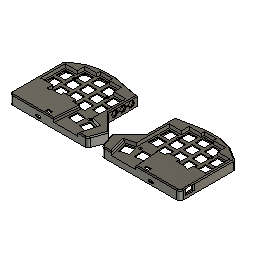
top_23332_2 (Autodesk Fusion 360 design; units mm, degrees)
Autodesk Fusion 360 part; units mm, degrees
note: some values were not read from the file. Set by a fixed rule: which sketch regions a step uses.
sketch "case_plate_23332_2" plane through (0, 0, 0) normal (0, 0, 1) x (1, 0, 0)
  line L0 (-131.5, 89.0512) -> (-131.5, 7.28)
  line L1 (-131.5, 7.28) -> (-13.7052, 7.28)
  line L2 (-32.5, 98.826) -> (-72.3112, 106.482)
  line L3 (-91.6231, 106.5) -> (-111.8983, 101.4312)
  line L4 (-13.7052, 7.28) -> (-6.0652, 28.2707)
  line L5 (-72.3112, 106.482) -> (-72.4047, 106.5)
  line L6 (-72.4047, 106.5) -> (-91.6231, 106.5)
  line L7 (-6.0652, 28.2707) -> (-32.5, 54.6647)
  line L8 (-32.5, 54.6647) -> (-32.5, 98.826)
  line L9 (-111.8983, 101.4312) -> (-131.5, 89.0512)
  line L10 (-29.5, 101.3041) -> (-72.1189, 109.5)
  line L11 (-91.9924, 109.5) -> (-113.0931, 104.2248)
  line L12 (-2.5919, 29.0421) -> (-29.5, 55.9087)
  line L13 (-134.5, 90.7047) -> (-134.5, 4.28)
  line L14 (-11.6046, 4.28) -> (-2.5919, 29.0421)
  line L15 (-134.5, 4.28) -> (-11.6046, 4.28)
  line L16 (-72.1189, 109.5) -> (-91.9924, 109.5)
  line L17 (-113.0931, 104.2248) -> (-134.5, 90.7047)
  line L18 (-29.5, 55.9087) -> (-29.5, 101.3041)
  line L19 (-112.3762, 102.5487) -> (-132.7, 89.7126)
  line L20 (-12.865, 6.08) -> (-4.6759, 28.5793)
  line L21 (-31.3, 99.8172) -> (-72.2904, 107.7)
  line L22 (-4.6759, 28.5793) -> (-31.3, 55.1623)
  line L23 (-91.7708, 107.7) -> (-112.3762, 102.5487)
  line L24 (-132.7, 89.7126) -> (-132.7, 6.08)
  line L25 (-31.3, 55.1623) -> (-31.3, 99.8172)
  line L26 (-132.7, 6.08) -> (-12.865, 6.08)
  line L27 (-72.2904, 107.7) -> (-91.7708, 107.7)
  line L28 (-12.4448, 5.48) -> (-3.9812, 28.7336)
  line L29 (-112.6152, 103.1074) -> (-133.3, 90.0433)
  line L30 (-133.3, 90.0433) -> (-133.3, 5.48)
  line L31 (-91.8447, 108.3) -> (-112.6152, 103.1074)
  line L32 (-72.2332, 108.3) -> (-91.8447, 108.3)
  line L33 (-30.7, 100.3128) -> (-71.9712, 108.2496)
  line L34 (-133.3, 5.48) -> (-12.4448, 5.48)
  line L35 (-3.9812, 28.7336) -> (-30.7, 55.4111)
  line L36 (-30.7, 55.4111) -> (-30.7, 100.3128)
  line L37 (-71.9712, 108.2496) -> (-72.2332, 108.3)
  circle A0 centre (-108, 80.5) radius 2.2
  circle A1 centre (-56, 80.5) radius 2.2
  circle A2 centre (-39.8644, 36.6759) radius 2.2
  line L38 (-96.5, 10.39) -> (-96.5, 28.39)
  line L39 (-96.5, 28.39) -> (-129.5, 28.39)
  line L40 (-129.5, 10.39) -> (-96.5, 10.39)
  line L41 (-129.5, 28.39) -> (-129.5, 10.39)
  line L42 (-92.975, 13.01) -> (-92.975, 7.16)
  line L43 (-84.175, 7.16) -> (-84.175, 13.01)
  line L44 (-84.175, 13.01) -> (-92.975, 13.01)
  line L45 (-82.175, 12.025) -> (-82.175, 8.525)
  line L46 (-73.175, 8.525) -> (-73.175, 12.025)
  line L47 (-73.175, 12.025) -> (-82.175, 12.025)
  line L48 (-82.175, 8.525) -> (-73.175, 8.525)
  line L49 (-17.3936, 37.8282) -> (-25.1718, 45.6064)
  line L50 (-25.1718, 45.6064) -> (-31.6064, 39.1718)
  line L51 (-21.0041, 34.2177) -> (-17.3936, 37.8282)
  line L52 (-96.8, 31.55) -> (-96.8, 40.45)
  line L53 (-96.8, 40.45) -> (-104.8004, 40.45)
  line L54 (-105.4, 39.7287) -> (-105.4, 31.55)
  line L55 (-105.4, 31.55) -> (-96.8, 31.55)
  line L56 (-127, 52) -> (-113, 52)
  line L57 (-113, 66) -> (-127, 66)
  line L58 (-127, 66) -> (-127, 52)
  line L59 (-113, 52) -> (-113, 66)
  line L60 (-127, 71) -> (-113, 71)
  line L61 (-113, 71) -> (-113, 85)
  line L62 (-127, 85) -> (-127, 71)
  line L63 (-113, 85) -> (-127, 85)
  line L64 (-108, 59) -> (-108, 45)
  line L65 (-94, 45) -> (-94, 59)
  line L66 (-94, 59) -> (-108, 59)
  line L67 (-108, 45) -> (-94, 45)
  line L68 (-94, 64) -> (-94, 78)
  line L69 (-94, 78) -> (-108, 78)
  line L70 (-108, 78) -> (-108, 64)
  line L71 (-108, 64) -> (-94, 64)
  line L72 (-108, 83) -> (-94, 83)
  line L73 (-94, 83) -> (-94, 97)
  line L74 (-108, 97) -> (-108, 83)
  line L75 (-94, 97) -> (-108, 97)
  line L76 (-89, 50) -> (-75, 50)
  line L77 (-75, 64) -> (-89, 64)
  line L78 (-75, 50) -> (-75, 64)
  line L79 (-89, 64) -> (-89, 50)
  line L80 (-89, 83) -> (-89, 69)
  line L81 (-89, 69) -> (-75, 69)
  line L82 (-75, 69) -> (-75, 83)
  line L83 (-75, 83) -> (-89, 83)
  line L84 (-75, 88) -> (-75, 102)
  line L85 (-75, 102) -> (-89, 102)
  line L86 (-89, 88) -> (-75, 88)
  line L87 (-89, 102) -> (-89, 88)
  line L88 (-70, 59) -> (-70, 45)
  line L89 (-56, 45) -> (-56, 59)
  line L90 (-70, 45) -> (-56, 45)
  line L91 (-56, 59) -> (-70, 59)
  line L92 (-70, 64) -> (-56, 64)
  line L93 (-56, 78) -> (-70, 78)
  line L94 (-70, 78) -> (-70, 64)
  line L95 (-56, 64) -> (-56, 78)
  line L96 (-56, 97) -> (-70, 97)
  line L97 (-70, 83) -> (-56, 83)
  line L98 (-70, 97) -> (-70, 83)
  line L99 (-56, 83) -> (-56, 97)
  line L100 (-37, 66) -> (-51, 66)
  line L101 (-51, 52) -> (-37, 52)
  line L102 (-37, 52) -> (-37, 66)
  line L103 (-51, 66) -> (-51, 52)
  line L104 (-51, 71) -> (-37, 71)
  line L105 (-51, 85) -> (-51, 71)
  line L106 (-37, 71) -> (-37, 85)
  line L107 (-37, 85) -> (-51, 85)
  line L108 (-59.7995, 22.3659) -> (-45.8527, 21.1457)
  line L109 (-45.8527, 21.1457) -> (-44.6325, 35.0924)
  line L110 (-58.5793, 36.3126) -> (-59.7995, 22.3659)
  line L111 (-44.6325, 35.0924) -> (-58.5793, 36.3126)
  line L112 (-35.9254, 33.5571) -> (-39.5489, 20.0342)
  line L113 (-39.5489, 20.0342) -> (-26.0259, 16.4107)
  line L114 (-26.0259, 16.4107) -> (-22.4025, 29.9337)
  line L115 (-22.4025, 29.9337) -> (-35.9254, 33.5571)
  line L116 (-131.5, 49.25) -> (-110.75, 49.25)
  line L117 (-129.75, 49.25) -> (-129.75, 87.75)
  line L118 (-110.75, 87.75) -> (-129.75, 87.75)
  line L119 (-91.25, 42.25) -> (-91.25, 47.25)
  line L120 (-110.75, 49.25) -> (-110.75, 42.25)
  line L121 (-91.75, 99.75) -> (-110.75, 99.75)
  line L122 (-110.75, 99.75) -> (-110.75, 87.75)
  line L123 (-91.25, 47.25) -> (-72.75, 47.25)
  line L124 (-72.25, 99.75) -> (-72.25, 104.75)
  line L125 (-72.25, 104.75) -> (-91.75, 104.75)
  line L126 (-91.75, 104.75) -> (-91.75, 99.75)
  line L127 (-72.75, 42.25) -> (-60.8203, 42.25)
  line L128 (-72.75, 47.25) -> (-72.75, 42.25)
  line L129 (-53.25, 87.75) -> (-53.25, 99.75)
  line L130 (-53.25, 99.75) -> (-72.25, 99.75)
  line L131 (-34.25, 54.6647) -> (-34.25, 87.75)
  line L132 (-34.25, 87.75) -> (-53.25, 87.75)
  line L133 (-62.7787, 19.866) -> (-43.1315, 18.1471)
  line L134 (-64.1423, 4.28) -> (-60.8203, 42.25)
  line L135 (-43.1315, 18.1471) -> (-24.0814, 13.0427)
  line L136 (-26.4293, 4.28) -> (-19.0344, 31.8782)
  line L137 (-34.25, 35.9552) -> (-6.2465, 28.4517)
  line L138 (-32.5, 54.6647) -> (-34.25, 54.6647)
  arc A3 (-108, 40.3) -> (-105.8143, 42.25) centre (-108, 42.5) ccw
  line L139 (-105.8143, 42.25) -> (-91.25, 42.25)
  line L140 (-131.5, 47.65) -> (-112.35, 47.65)
  line L141 (-112.35, 47.65) -> (-112.35, 40.65)
  line L142 (-104.6807, 40.65) -> (-89.65, 40.65)
  line L143 (-89.65, 40.65) -> (-89.65, 45.65)
  line L144 (-89.65, 45.65) -> (-74.35, 45.65)
  line L145 (-74.35, 45.65) -> (-74.35, 40.65)
  line L146 (-74.35, 40.65) -> (-62.5664, 40.65)
  line L147 (-34.25, 35.9552) -> (-34.25, 54.6647)
  line L148 (-32.5, 37.298) -> (-32.5, 54.6647)
  line L149 (-65.4859, 7.28) -> (-62.5664, 40.65)
  line L150 (-32.5, 37.298) -> (-8.7266, 30.928)
  line L151 (-31.6064, 39.1718) -> (-28.7198, 36.2851)
  line L152 (-108, 40.3) -> (-110.75, 40.3)
  line L153 (-110.75, 40.3) -> (-110.75, 42.25)
  line L154 (-65.7484, 4.28) -> (-62.5664, 40.65)
  line L155 (-74.35, 40.65) -> (-62.5664, 40.65)
  line L156 (-74.35, 45.65) -> (-74.35, 40.65)
  line L157 (-89.65, 45.65) -> (-74.35, 45.65)
  line L158 (-89.65, 40.65) -> (-89.65, 45.65)
  line L159 (-104.6807, 40.65) -> (-89.65, 40.65)
  arc A4 (-108, 38.7) -> (-104.6807, 40.65) centre (-108, 42.5) ccw
  line L160 (-108, 38.7) -> (-112.35, 38.7)
  line L161 (-112.35, 38.7) -> (-112.35, 42.25)
  line L162 (-112.35, 47.65) -> (-112.35, 42.25)
  line L163 (-131.5, 47.65) -> (-112.35, 47.65)
  constraint coincident L15 L154.start
extrude "Extrude1" add sketch "case_plate_23332_2" against normal blind 6.8 contours L0 L1 L2 L3 L4 L5 L6 L7 L8 L9 L19 L20 L21 L22 L23 L24 L25 L26 L27 L136 L154 | L1 L26 L134 L154 | L1 L26 L134 L136 | L19 L20 L21 L22 L23 L24 L25 L26 L27 L28 L29 L30 L31 L32 L33 L34 L35 L36 L37 L136 L154 | L26 L34 L134 L154 | L26 L34 L134 L136 makes body 1
extrude "Extrude2" add sketch "case_plate_23332_2" against normal blind 7.6 contours L10 L11 L12 L13 L14 L15 L16 L17 L18 L28 L29 L30 L31 L32 L33 L34 L35 L36 L37 L136 L154 | L15 L34 L134 L154 | L15 L34 L134 L136 bodies 1
extrude "Extrude3" add sketch "case_plate_23332_2" along normal blind 1.6 contours L116 L117 L118 L119 L120 L121 L122 L123 L124 L125 L126 L127 L128 L129 L130 L131 L132 L133 L134 L135 L136 L137 A3 L139 L147 L152 L153 | L1 L133 L134 L135 L136 | L1 L26 L134 L136 | L26 L34 L134 L136 | L15 L34 L134 L136 | A0 | A1 | A2 bodies 1
extrude "Extrude4" add sketch "case_plate_23332_2" along normal blind 7 contours L0 L2 L3 L5 L6 L8 L9 L116 L117 L118 L121 L122 L124 L125 L126 L129 L130 L131 L132 L138 | L0 L1 L2 L3 L4 L5 L6 L7 L8 L9 L19 L20 L21 L22 L23 L24 L25 L26 L27 L136 L154 | L0 L1 L116 L119 L120 L123 L127 L128 L134 A3 L139 L140 L141 L142 L143 L144 L145 L146 L149 L152 L153 L154 L155 L156 L157 L158 L159 A4 L160 L161 L162 L163 | L1 L26 L134 L154 | L7 L137 L138 L147 L148 L150 | L19 L20 L21 L22 L23 L24 L25 L26 L27 L28 L29 L30 L31 L32 L33 L34 L35 L36 L37 L136 L154 | L26 L34 L134 L154 | L1 L4 L7 L136 L137 | L10 L11 L12 L13 L14 L15 L16 L17 L18 L28 L29 L30 L31 L32 L33 L34 L35 L36 L37 L136 L154 | L15 L34 L134 L154 bodies 1
extrude "Extrude5" add sketch "case_plate_23332_2" along normal blind 1.6 from surface at 5.4 contours L0 L1 L42 L43 L44 L52 L53 L54 L55 L140 L141 L142 L143 L144 L145 L146 L149 L154 L155 L156 L157 L158 L159 A4 L160 L161 L162 L163 | L1 L42 L43 L44 | L7 L49 L50 L51 L148 L150 L151 | L52 L53 L54 L55 A4 | L49 L50 L51 L150 L151 | L38 L39 L40 L41 | L45 L46 L47 L48 bodies 1
move_body "Move1" bodies 1 to x (1, 0, 0) y (0, 1, 0) z (0, 0, 1) at (0, 0, -1.6)
hole "Hole1" at (-108, 80.5, 0) at (-108, 42.5, 0) at (-56, 80.5, 0) at (-39.8644, 36.6759, 0) direction (0, 0, -1) diameter 2.4 depth 1.6 tip angle 118 countersink diameter 4.4 countersink angle 90 bodies 1
sketch "usb" plane through (-134.5, 0, 0) normal (-1, 0, 0) x (0, -1, 0)
  line L0 (-90.7047, 5.4) -> (-90.7047, -9.2)
  line L1 (-90.7047, -9.2) -> (-4.28, -9.2)
  line L2 (-4.28, -9.2) -> (-4.28, 5.4)
  line L3 (-4.28, 5.4) -> (-90.7047, 5.4)
  line L4 (-28.39, 0) -> (-10.39, 0)
  line L5 (-28.0836, 4.2) -> (-9.5388, 4.2)
  line L6 (-28.0154, -3.8) -> (-9.9886, -3.8)
  line L7 (-25.39, 4.2) -> (-25.39, -3.8)
  line L8 (-13.39, 4.2) -> (-13.39, -3.8)
  dimension "d17" = 1.2
  dimension "d18" = 8
  dimension "d19" = 12
  dimension "d20" = 3
  constraint parallel L3 L5
  constraint parallel L4 L6
  constraint coincident L5 L7.start
  constraint coincident L6 L7.end
  constraint perpendicular L6 L7
  constraint coincident L5 L8.start
  constraint coincident L6 L8.end
  constraint perpendicular L6 L8
  measures "d17" distance of L3 L5
  measures "d18" distance of L5 L6
  measures "d19" distance of L7 L8
  measures "d20" distance of L4.start L7
extrude "Extrude6" cut sketch "usb" against normal up to surface (3 mm away) contours L4 L5 L7 L8 | L4 L6 L7 L8 bodies 1
sketch "vik" plane through (13.2271, 13.2476, 0) normal (0.70656, 0.707653, 0) x (-0.707653, 0.70656, 0)
  line L0 (22.3542, 5.4) -> (22.3542, -9.2)
  line L1 (22.3542, -9.2) -> (60.3786, -9.2)
  line L2 (60.3786, -9.2) -> (60.3786, 5.4)
  line L3 (60.3786, 5.4) -> (22.3542, 5.4)
  line L4 (39.0366, 0) -> (50.0365, 0)
  line L5 (39.0366, 0) -> (39.0366, -5) construction
  line L6 (50.0365, 0) -> (50.0365, -5) construction
  line L7 (36.4982, -5) -> (39.0366, -5) construction
  line L8 (50.0365, -5) -> (52.593, -5) construction
  line L9 (39.0366, -5) -> (50.0365, -5) construction
  line L10 (39.0366, -5.5) -> (50.0365, -5.5) construction
  line L11 (39.0366, -4.5) -> (50.0365, -4.5) construction
  line L12 (41.0366, -4.5) -> (41.0366, -5.5)
  line L13 (48.0366, -4.5) -> (48.0366, -5.5)
  line L14 (41.0366, -4.5) -> (48.0366, -4.5)
  line L15 (48.0366, -4.5) -> (48.0366, -5.5)
  line L16 (48.0366, -5.5) -> (41.0366, -5.5)
  line L17 (41.0366, -5.5) -> (41.0366, -4.5)
  dimension "d23" = 10.4
  dimension "d24" = 0.5
  dimension "d25" = -0.5
  dimension "d26" = 7
  dimension "d27" = 2
  constraint horizontal L7
  constraint coincident L4.start L5.start
  constraint perpendicular L5 L7
  constraint coincident L4.end L6.start
  constraint coincident L6.end L7
  constraint perpendicular L6 L7
  constraint coincident L11 L12.start
  constraint coincident L10 L12.end
  constraint perpendicular L10 L12
  constraint coincident L11 L13.start
  constraint coincident L10 L13.end
  constraint perpendicular L10 L13
  constraint horizontal L14
  constraint vertical L15
  constraint horizontal L16
  constraint vertical L17
  measures "d23" distance of L3 L7
  measures "d26" distance of L12 L13
  measures "d27" distance of L5.end L12
extrude "Extrude7" cut sketch "vik" against normal up to surface (3 mm away) contours L12 L13 L14 L15 L16 L17 bodies 1
sketch "rst" plane through (0, 0, 5.4) normal (0, 0, 1) x (-1, 0, 0)
  line L0 (108, -40.3) -> (110.75, -40.3)
  line L1 (110.75, -40.3) -> (110.75, -49.25)
  line L2 (110.75, -49.25) -> (129.75, -49.25)
  line L3 (129.75, -49.25) -> (129.75, -87.75)
  line L4 (129.75, -87.75) -> (110.75, -87.75)
  line L5 (110.75, -87.75) -> (110.75, -99.75)
  line L6 (110.75, -99.75) -> (91.75, -99.75)
  line L7 (91.75, -99.75) -> (91.75, -104.75)
  line L8 (91.75, -104.75) -> (72.25, -104.75)
  line L9 (72.25, -104.75) -> (72.25, -99.75)
  line L10 (72.25, -99.75) -> (53.25, -99.75)
  line L11 (53.25, -99.75) -> (53.25, -87.75)
  line L12 (53.25, -87.75) -> (34.25, -87.75)
  line L13 (34.25, -87.75) -> (34.25, -35.9552)
  line L14 (34.25, -35.9552) -> (19.0344, -31.8782)
  line L15 (19.0344, -31.8782) -> (26.4293, -4.28)
  line L16 (26.4293, -4.28) -> (11.6046, -4.28)
  line L17 (11.6046, -4.28) -> (2.5919, -29.0421)
  line L18 (2.5919, -29.0421) -> (29.5, -55.9087)
  line L19 (29.5, -55.9087) -> (29.5, -101.3041)
  line L20 (29.5, -101.3041) -> (72.1189, -109.5)
  line L21 (72.1189, -109.5) -> (91.9924, -109.5)
  line L22 (91.9924, -109.5) -> (113.0931, -104.2248)
  line L23 (113.0931, -104.2248) -> (134.5, -90.7047)
  line L24 (134.5, -90.7047) -> (134.5, -4.28)
  line L25 (134.5, -4.28) -> (64.1423, -4.28)
  line L26 (64.1423, -4.28) -> (60.8203, -42.25)
  line L27 (60.8203, -42.25) -> (72.75, -42.25)
  line L28 (72.75, -42.25) -> (72.75, -47.25)
  line L29 (72.75, -47.25) -> (91.25, -47.25)
  line L30 (91.25, -47.25) -> (91.25, -42.25)
  line L31 (91.25, -42.25) -> (105.8143, -42.25)
  arc A0 (108, -40.3) -> (105.8143, -42.25) centre (108, -42.5) ccw
  line L32 (73.175, -8.525) -> (73.175, -12.025)
  line L33 (73.175, -12.025) -> (82.175, -12.025)
  line L34 (82.175, -12.025) -> (82.175, -8.525)
  line L35 (82.175, -8.525) -> (73.175, -8.525)
  line L36 (80.675, -12.025) -> (80.675, -8.525)
  line L37 (74.675, -12.025) -> (74.675, -8.525)
  dimension "d30" = 6
  dimension "d31" = 1.5
  constraint coincident L33 L36.start
  constraint coincident L35 L36.end
  constraint perpendicular L35 L36
  constraint coincident L33 L37.start
  constraint coincident L35 L37.end
  constraint perpendicular L35 L37
  measures "d30" distance of L36 L37
  measures "d31" distance of L34 L36
extrude "Extrude8" cut sketch "rst" against normal up to surface (1.6 mm away) contours L33 L35 L36 L37 bodies 1
sketch "pwr" plane through (0, 4.28, 0) normal (0, -1, 0) x (1, 0, 0)
  line L0 (-134.5, 5.4) -> (-134.5, -7.2)
  line L1 (-134.5, -7.2) -> (-11.6046, -7.2)
  line L2 (-11.6046, -7.2) -> (-11.6046, 5.4)
  line L3 (-11.6046, 5.4) -> (-26.4293, 5.4)
  line L4 (-26.4293, 5.4) -> (-26.4293, 0)
  line L5 (-26.4293, 0) -> (-64.1423, 0)
  line L6 (-64.1423, 0) -> (-64.1423, 5.4)
  line L7 (-64.1423, 5.4) -> (-134.5, 5.4)
  line L8 (-84.175, 0) -> (-92.975, 0)
  line L9 (-95.0802, -5) -> (-79.921, -5) construction
  line L10 (-94.9804, -4.25) -> (-79.5417, -4.25) construction
  line L11 (-90.575, 0) -> (-90.575, -4.25) construction
  line L12 (-86.575, 0) -> (-86.575, -4.25) construction
  line L13 (-90.575, -5.75) -> (-86.575, -5.75)
  arc A0 (-86.575, -5.75) -> (-86.575, -2.75) centre (-86.575, -4.25) ccw
  line L14 (-86.575, -2.75) -> (-90.575, -2.75)
  arc A1 (-90.575, -2.75) -> (-90.575, -5.75) centre (-90.575, -4.25) ccw
  line L15 (-90.575, -4.25) -> (-86.575, -4.25) construction
  line L16 (-134.5, 5.4) -> (-134.5, -7.2)
  line L17 (-134.5, -7.2) -> (-11.6046, -7.2)
  line L18 (-11.6046, -7.2) -> (-11.6046, 5.4)
  line L19 (-11.6046, 5.4) -> (-26.4293, 5.4)
  line L20 (-26.4293, 5.4) -> (-26.4293, 0)
  line L21 (-26.4293, 0) -> (-64.1423, 0)
  line L22 (-64.1423, 0) -> (-64.1423, 5.4)
  line L23 (-64.1423, 5.4) -> (-134.5, 5.4)
  line L24 (-134.5, 5.4) -> (-134.5, -9.2)
  line L25 (-134.5, -9.2) -> (-11.6046, -9.2)
  line L26 (-11.6046, -9.2) -> (-11.6046, 5.4)
  line L27 (-11.6046, 5.4) -> (-26.4293, 5.4)
  line L28 (-26.4293, 5.4) -> (-26.4293, 0)
  line L29 (-26.4293, 0) -> (-64.1423, 0)
  line L30 (-64.1423, 0) -> (-64.1423, 5.4)
  line L31 (-64.1423, 5.4) -> (-134.5, 5.4)
  line L32 (-134.5, 5.4) -> (-134.5, -9.2)
  line L33 (-134.5, -9.2) -> (-11.6046, -9.2)
  line L34 (-11.6046, -9.2) -> (-11.6046, 5.4)
  line L35 (-11.6046, 5.4) -> (-26.4293, 5.4)
  line L36 (-26.4293, 5.4) -> (-26.4293, 0)
  line L37 (-26.4293, 0) -> (-64.1423, 0)
  line L38 (-64.1423, 0) -> (-64.1423, 5.4)
  line L39 (-64.1423, 5.4) -> (-134.5, 5.4)
  dimension "d34" = 10.4
  dimension "d35" = 0.75
  dimension "d36" = 4
  dimension "d37" = 2.4
  dimension "d38" = 3
  constraint parallel L7 L9
  constraint horizontal L10
  constraint coincident L8 L11.start
  constraint coincident L10 L11.end
  constraint perpendicular L10 L11
  constraint coincident L8 L12.start
  constraint coincident L10 L12.end
  constraint perpendicular L10 L12
  constraint tangent L13 A0
  constraint tangent A0 L14
  constraint parallel L13 L14
  constraint tangent L14 A1
  constraint tangent L13 A1
  constraint coincident L12.end A0.centre
  constraint perpendicular L12 L15
  constraint coincident L11.end A1.centre
  measures "d34" distance of L7 L9
  measures "d35" distance of L9 L10
  measures "d36" distance of L11 L12
  measures "d37" distance of L8.end L11
  measures "d38" diameter of A0
extrude "Extrude11" cut sketch "pwr" along normal up to surface (-3 mm away) and the other way blind -1 contours L13 A0 L14 A1 bodies 1
sketch "Sketch7" plane through (0, 0, -5.75) normal (0, 0, 1) x (-1, 0, 0)
  line L0 (90.575, -4.28) -> (86.575, -4.28)
  line L1 (86.575, -4.28) -> (86.575, -7.28)
  line L2 (86.575, -7.28) -> (90.575, -7.28)
  line L3 (90.575, -7.28) -> (90.575, -4.28)
  line L4 (90.575, -5.78) -> (86.575, -5.78)
  constraint midpoint L3 L4.start
  constraint midpoint L1 L4.end
extrude "Extrude12" cut sketch "Sketch7" against normal up to surface (2.65 mm away) contours L1 L2 L3 L4 bodies 1
sketch "Sketch8" plane through (-29.5, 0, 0) normal (1, 0, 0) x (0, 1, 0)
  line L0 (55.9087, 5.4) -> (55.9087, -9.2)
  line L1 (55.9087, -9.2) -> (101.3041, -9.2)
  line L2 (101.3041, -9.2) -> (101.3041, 5.4)
  line L3 (101.3041, 5.4) -> (55.9087, 5.4)
  line L4 (55.9087, -1.5) -> (101.3041, -1.5) construction
  line L5 (80.9066, 2.472) -> (76.3166, 2.478)
  line L6 (76.3166, 2.478) -> (74.0164, -1.4939)
  line L7 (74.0164, -1.4939) -> (76.3062, -5.472)
  line L8 (76.3062, -5.472) -> (80.8961, -5.478)
  line L9 (80.8961, -5.478) -> (83.1963, -1.5061)
  line L10 (83.1963, -1.5061) -> (80.9066, 2.472)
  line L11 (87.0164, -1.5061) -> (89.3166, -5.478)
  line L12 (89.3166, -5.478) -> (93.9066, -5.472)
  line L13 (93.9066, -5.472) -> (96.1963, -1.4939)
  line L14 (96.1963, -1.4939) -> (93.8961, 2.478)
  line L15 (93.8961, 2.478) -> (89.3062, 2.472)
  line L16 (89.3062, 2.472) -> (87.0164, -1.5061)
  line L17 (67.8961, 2.478) -> (63.3062, 2.472)
  line L18 (63.3062, 2.472) -> (61.0164, -1.5061)
  line L19 (61.0164, -1.5061) -> (63.3166, -5.478)
  line L20 (63.3166, -5.478) -> (67.9066, -5.472)
  line L21 (67.9066, -5.472) -> (70.1963, -1.4939)
  line L22 (70.1963, -1.4939) -> (67.8961, 2.478)
  line L23 (66.3564, -2.25) -> (90.8564, -2.25)
  arc A0 (90.8564, -2.25) -> (90.8564, -0.75) centre (90.8564, -1.5) ccw
  line L24 (90.8564, -0.75) -> (66.3564, -0.75)
  arc A1 (66.3564, -0.75) -> (66.3564, -2.25) centre (66.3564, -1.5) ccw
  line L25 (65.6064, -1.5) -> (91.6064, -1.5) construction
  point P0 (65.6064, -1.5)
  point P1 (78.6064, -1.5)
  point P2 (91.6064, -1.5)
  point P3 (78.6064, -1.5)
  point P4 (91.6064, -1.5)
  point P5 (65.6064, -1.5)
  dimension "d51" = 6.9
  dimension "d52" = 13
  dimension "d53" = 13
  dimension "d54" = 3.975
  dimension "d55" = 3.975
  dimension "d56" = 3.975
  dimension "d57" = 1.5
  constraint coincident L0 L4.start
  constraint coincident L2 L4.end
  constraint perpendicular L2 L4
  constraint coincident L4 P5
  constraint coincident L4 P3
  constraint midpoint L4 P3
  constraint coincident L4 P4
  constraint coincident P3 P1
  constraint coincident P4 P2
  constraint coincident P5 P0
  constraint tangent L23 A0
  constraint tangent A0 L24
  constraint parallel L23 L24
  constraint tangent L24 A1
  constraint tangent L23 A1
  constraint midpoint A1 P5
  constraint midpoint A0 P4
  constraint parallel L4 L25
  measures "d51" distance of L3 L4
  measures "d52" distance of P5 P3
  measures "d53" distance of P3 P4
  measures "d54" distance of P3 L10
  measures "d55" distance of P4 L16
  measures "d56" distance of P5 L22
  measures "d57" diameter of A0
extrude "Extrude13" cut sketch "Sketch8" against normal blind 2 contours L5 L6 L10 L24 | L9 L10 L11 L16 L23 L24 | L6 L7 L9 L10 L23 L24 | L6 L7 L21 L22 L23 L24 | L11 L16 L23 A0 L24 | L11 L12 L13 L14 L15 L16 L23 A0 L24 | L17 L18 L19 L20 L21 L22 L23 L24 A1 | L21 L22 L23 L24 A1 | L7 L8 L9 L23 bodies 1
chamfer "Chamfer5" distance 0.4 angle 45 19 edges at (-29.5, 65.6011, 2.475) (-29.5, 62.1613, 0.483) (-29.5, 62.1665, -3.492) (-29.5, 65.6116, -5.475) (-29.5, 68.8338, -3.861) (-44, 66, 0) (-29.5, 75.3819, 0.864) (-29.5, 78.6116, 2.475) (-29.5, 75.3789, -3.861) (-29.5, 78.6011, -5.475) (-29.5, 81.8308, -3.864) (-29.5, 81.8338, 0.861) (-29.5, 88.3789, 0.861) (-29.5, 91.6011, 2.475) (-29.5, 95.0462, 0.492) (-29.5, 95.0514, -3.483) (-29.5, 91.6116, -5.475) (-29.5, 88.3819, -3.864) (-29.5, 68.8308, 0.864) on bodies 1
sketch "Sketch9" plane through (13.2271, 13.2476, 0) normal (0.70656, 0.707653, 0) x (-0.707653, 0.70656, 0)
  line L0 (41.0366, -5.5) -> (41.0366, -4.5)
  line L1 (41.0366, -4.5) -> (48.0366, -4.5)
  line L2 (48.0366, -4.5) -> (48.0366, -5.5)
  line L3 (48.0366, -5.5) -> (41.0366, -5.5)
  line L4 (22.3542, 5.4) -> (22.3542, -9.2)
  line L5 (22.3542, -9.2) -> (60.3786, -9.2)
  line L6 (60.3786, -9.2) -> (60.3786, 5.4)
  line L7 (60.3786, 5.4) -> (22.3542, 5.4)
  line L8 (22.3542, -1.5) -> (60.3786, -1.5) construction
  line L9 (54.695, 2.4626) -> (50.1051, 2.4873)
  line L10 (50.1051, 2.4873) -> (47.7887, -1.4752)
  line L11 (47.7887, -1.4752) -> (50.0622, -5.4626)
  line L12 (50.0622, -5.4626) -> (54.6521, -5.4873)
  line L13 (54.6521, -5.4873) -> (56.9685, -1.5248)
  line L14 (56.9685, -1.5248) -> (54.695, 2.4626)
  line L15 (35.1042, -2.25) -> (51.6286, -2.25)
  arc A0 (51.6286, -2.25) -> (51.6286, -0.75) centre (51.6286, -1.5) ccw
  line L16 (51.6286, -0.75) -> (35.1042, -0.75)
  arc A1 (35.1042, -0.75) -> (35.1042, -2.25) centre (35.1042, -1.5) ccw
  line L17 (34.3542, -1.5) -> (52.3786, -1.5) construction
  line L18 (36.6614, 2.4679) -> (32.0715, 2.4821)
  line L19 (32.0715, 2.4821) -> (29.7643, -1.4858)
  line L20 (29.7643, -1.4858) -> (32.047, -5.4679)
  line L21 (32.047, -5.4679) -> (36.6369, -5.4821)
  line L22 (36.6369, -5.4821) -> (38.9441, -1.5142)
  line L23 (38.9441, -1.5142) -> (36.6614, 2.4679)
  point P0 (52.3786, -1.5)
  point P1 (52.3786, -1.5)
  point P2 (34.3542, -1.5)
  point P3 (34.3542, -1.5)
  point P4 (34.3542, -1.5)
  dimension "d60" = 6.9
  dimension "d61" = 3.975
  dimension "d62" = 8
  dimension "d66" = 12
  dimension "d67" = 1.5
  dimension "d87" = 3.975
  constraint coincident L4 L8.start
  constraint coincident L6 L8.end
  constraint perpendicular L6 L8
  constraint coincident L8 P1
  constraint coincident P1 P0
  constraint coincident L8 P4
  constraint coincident P4 P3
  constraint tangent L15 A0
  constraint tangent A0 L16
  constraint parallel L15 L16
  constraint tangent L16 A1
  constraint tangent L15 A1
  constraint midpoint A1 P4
  constraint midpoint A0 P1
  constraint parallel L8 L17
  measures "d60" distance of L7 L8
  measures "d61" distance of P1 L14
  measures "d62" distance of L8.end P1
  measures "d66" distance of L8.start P4
  measures "d67" diameter of A0
  measures "d87" distance of P4 L23
extrude "Extrude14" cut sketch "Sketch9" against normal blind 2 contours L9 L10 L11 L12 L13 L14 L15 A0 L16 | L10 L11 L15 A0 L16 | L10 L11 L15 L16 L22 L23 | L15 L16 A1 L22 L23 | L15 L16 A1 L18 L19 L20 L21 L22 L23 bodies 1
chamfer "Chamfer6" distance 0.4 angle 45 12 edges at (-21.5603, 47.9813, 0.8687) (-23.854, 50.2713, 2.4749) (-21.5515, 47.9724, -3.8563) (-23.8236, 50.241, -5.4749) (-26.2672, 52.6809, -3.5061) (-26.2824, 52.696, 0.4689) (-13.3692, 39.8027, 0.859) (-11.0924, 37.5295, 2.475) (-8.652, 35.0929, 0.4981) (-8.6434, 35.0842, -3.4769) (-11.0751, 37.5122, -5.475) (-13.3641, 39.7977, -3.866) on bodies 1
fillet "Fillet1" radius 5 12 edges at (-11.6046, 4.28, -1.9) (-134.5, 4.28, -1.9) (-134.5, 90.7047, -1.9) (-113.0931, 104.2248, -1.9) (-91.9924, 109.5, -1.9) (-72.1189, 109.5, -1.9) (-72.2332, 108.3, -8.8) (-91.8447, 108.3, -8.8) (-112.6152, 103.1074, -8.8) (-133.3, 90.0433, -8.8) (-133.3, 5.48, -8.8) (-12.4448, 5.48, -8.8) on bodies 1
fillet "Fillet1" radius 2 6 edges at (-72.4047, 106.5, -5) (-91.6231, 106.5, -5) (-111.8983, 101.4312, -5) (-131.5, 89.0512, -5) (-131.5, 7.28, -2.3) (-13.7052, 7.28, -5) on bodies 1
chamfer "Chamfer1" distance 1.5 angle 45 18 edges at (-62.4813, 23.265, 5.4) (-96.8211, 4.28, 5.4) (-50.5755, 105.357, 5.4) (-72.121, 109.4775, 5.4) (-81.9861, 109.5, 5.4) (-91.9878, 109.4625, 5.4) (-102.452, 106.8851, 5.4) (-113.0679, 104.166, 5.4) (-122.9708, 97.9863, 5.4) (-133.8789, 90.3624, 5.4) (-134.5, 48.6144, 5.4) (-133.0355, 5.7445, 5.4) (-29.5, 78.6064, 5.4) (-16.046, 42.4754, 5.4) (-6.4995, 18.306, 5.4) (-20.7675, 4.28, 5.4) (-12.2377, 5.1843, 5.4) (-22.7319, 18.0791, 5.4) on bodies 1
chamfer "Chamfer2" distance 0.4 angle 45 4 edges at (-74.675, 10.275, 5.4) (-77.675, 8.525, 5.4) (-80.675, 10.275, 5.4) (-77.675, 12.025, 5.4) on bodies 1
chamfer "Chamfer3" distance 0.5 angle 45 4 edges at (-88.575, 4.28, -2.75) (-85.075, 4.28, -4.25) (-88.575, 4.28, -5.75) (-92.075, 4.28, -4.25) on bodies 1
chamfer "Chamfer4" distance 1 angle 45 3 edges at (-134.5, 19.39, -3.8) (-134.5, 25.39, 0.05) (-134.5, 13.39, 0.05) on bodies 1
mirror "Mirror1" about plane through (0, 0, 0) normal (1, 0, 0) of bodies 1 makes body 2
